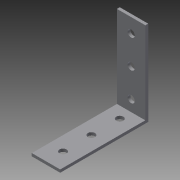
# Autodesk Inventor part: L-Gusset long
Saved by Autodesk Inventor 2015 (Build 190159000, 159)
## iProperties
Created: 2015-01-30
Part Number: L-Gusset long
Material: Generic
Document SubType Name: Modeling
Designer: chapale16
Density: 1 g/cm^3
Appearance: Default
Author: chapale16
Autodesk Inventor part; units mm, degrees
ref_plane "YZ Plane" through (0, 0, 0) normal (1, 0, 0) x (0, 1, 0)
ref_plane "XZ Plane" through (0, 0, 0) normal (0, 1, 0) x (-1, 0, 0)
ref_plane "XY Plane" through (0, 0, 0) normal (0, 0, 1) x (1, 0, 0)
sketch "Sketch1" plane through (0, 0, 0) normal (0, 0, 1) x (1, 0, 0)
  line L0 (0, 0) -> (0, 76.2)
  line L1 (0, 76.2) -> (-25.4, 76.2)
  line L2 (-25.4, 76.2) -> (-25.4, 0)
  line L3 (-25.4, 0) -> (0, 0)
  dimension "d0" = 76.2
  dimension "d2" = 25.4
  constraints: 8 end point, 2 perpendicular, 1 horizontal, 1 vertical
  measures "d0" distance of L0.start L0.end
  measures "d2" distance of L0.end L1.end
extrude "Extrusion1" add sketch "Sketch1" along normal blind 2.54
sketch "Sketch2" plane through (0, 0, 2.54) normal (0, 0, 1) x (1, 0, 0)
  line L0 (-25.4, 0) -> (-25.4, 2.54)
  line L1 (-25.4, 76.2) -> (-25.4, 0) projected
  line L2 (-25.4, 2.54) -> (0, 2.54)
  line L3 (0, 0) -> (0, 76.2) projected
  line L4 (0, 0) -> (-25.4, 0)
  line L5 (-25.4, 0) -> (0, 0) projected
  dimension "d5" = 2.54
  constraints: 6 end point, 2 point on line, 1 collinear, 1 perpendicular
  measures "d5" distance of L0.start L0.end
extrude "Extrusion2" add sketch "Sketch2" along normal blind 76.2
hole "Hole1" at (-12.7, 2.54, 12.7) direction (0, -1, 0) diameter 6.35 end through all
pattern_linear "Rectangular Pattern1" count 3 spacing 25.4 along (0, 0, 1) of "Hole1"
hole "Hole2" at (-12.7, 12.7, 2.54) direction (0, 0, -1) diameter 6.35 end through all
pattern_linear "Rectangular Pattern2" count 3 spacing 25.4 along (0, 1, 0) of "Hole2"
body "Solid1"
